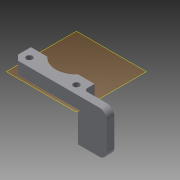
# Autodesk Inventor part: RightBracket
Saved by Autodesk Inventor 2014 SP1 (Build 180222100, 222)
## iProperties
Created: 2017-02-10
Part Number: RightBracket
Material: Generic
Document SubType Name: Modeling
Designer: danielsikar
Density: 1 g/cm^3
Appearance: Default
d0: 12.000 mm
d1: 12.000 mm
d2: 8.000 mm
d3: 0.00 deg
d4: 8.000 mm
d5: 5.000 mm
d6: 20.000 mm
d7: 0.00 deg
d8: 19.000 mm
d9: 5.000 mm
d10: 20.000 mm
d11: 0.00 deg
d14: 2.000 mm
d15: 0.500 mm
d16: 8.000 mm
d17: 0.00 deg
Author: danielsikar
Autodesk Inventor part; units mm, degrees
ref_plane "YZ Plane" through (0, 0, 0) normal (1, 0, 0) x (0, 1, 0)
ref_plane "XZ Plane" through (0, 0, 0) normal (0, 1, 0) x (-1, 0, 0)
ref_plane "XY Plane" through (0, 0, 0) normal (0, 0, 1) x (1, 0, 0)
ref_plane "Work Plane1" through (21, 21, 47) normal (0, 0, 1) x (1, 0, 0)
sketch "Sketch1" plane through (21, 21, 47) normal (0, 0, 1) x (1, 0, 0)
  line L0 (21, -17.5) -> (21, 17.5) construction
  line L1 (-17.5, -21) -> (17.5, -21) construction
  line L2 (21, -21) -> (9, -21)
  line L3 (9, -21) -> (9, -9)
  line L4 (9, -9) -> (21, -9)
  line L5 (21, -9) -> (21, -21)
  point P0 (-21, -21)
  dimension "d0" = 12
  dimension "d1" = 12
  constraints: 8 end point, 2 parallel, 1 horizontal, 1 perpendicular, 1 point on line
  measures "d0" distance of L3.end L4.end
  measures "d1" distance of L2.end L3.end
extrude "Extrusion1" add sketch "Sketch1" along normal blind 8
sketch "Sketch2" plane through (42, 0, 47) normal (1, 0, 0) x (0, 0, -1)
  line L0 (-8, 0) -> (0, 0)
  line L1 (0, 0) -> (0, 5)
  line L2 (0, 5) -> (-8, 5)
  line L3 (-8, 5) -> (-8, 0)
  point P0 (47, 0)
  dimension "d4" = 8
  dimension "d5" = 5
  constraints: 8 end point, 2 parallel, 1 horizontal, 1 perpendicular
  measures "d4" distance of L2.end L1.end
  measures "d5" distance of L1.end L0.end
extrude "Extrusion2" add sketch "Sketch2" along normal blind 20
sketch "Sketch3" plane through (21, 21, 47) normal (0, 0, -1) x (-1, 0, 0)
  line L0 (-41, -16) -> (-22, -16)
  line L1 (-22, -16) -> (-22, -21)
  line L2 (-22, -21) -> (-41, -21)
  line L3 (-41, -21) -> (-41, -16)
  point P0 (21, -21)
  dimension "d8" = 19
  dimension "d9" = 5
  constraints: 8 end point, 2 parallel, 1 horizontal, 1 perpendicular
  measures "d8" distance of L1.end L2.end
  measures "d9" distance of L0.end L1.end
extrude "Extrusion3" add sketch "Sketch3" along normal blind 20
fillet "Fillet3" radius 2 1 edges at (42, 5, 51)
sketch "Sketch4" plane through (21, 21, 55) normal (0, 0, 1) x (1, 0, 0)
  circle A0 centre (15.5, -15.5) radius 1.5 projected
  circle A1 centre (15.5, -15.5) radius 2
  point P0 (-21, -21)
  dimension "d15" = 0.5
  constraints: 1 centre point
  measures "d15" radial gap between concentric circles of A1 A0
extrude "Extrusion4" cut sketch "Sketch4" against normal blind 8 contours A0 | A1
sketch "Sketch5" plane through (30, 0, 47) normal (-1, 0, 0) x (0, 0, 1)
  line L0 (0, 0) -> (0, 12) projected
  line L1 (0, 0) -> (8, 0) projected
  line L2 (8, 12) -> (8, 0) projected
  line L3 (0, 12) -> (8, 12) projected
  point P0 (-47, 0)
ref_plane "Work Plane2" through (0, 3.5, 0) normal (-1, 0, 0) x (0, 0, 1)
extrude "Extrusion5" add sketch "Sketch5" along normal up to surface (30 mm away)
sketch "Sketch6" plane through (21, 21, 55) normal (0, 0, 1) x (1, 0, 0)
  circle A0 centre (-15.5, -15.5) radius 1.5 projected
  circle A1 centre (-15.5, -15.5) radius 2
  dimension "d20" = 0.5
  constraints: 1 centre point
  measures "d20" radial gap between concentric circles of A1 A0
extrude "Extrusion6" cut sketch "Sketch6" against normal blind 8 contours A0 | A1
sketch "Sketch7" plane through (21, 21, 55) normal (0, 0, 1) x (1, 0, 0)
  line L0 (21, -9) -> (-21, -9) projected
  circle A0 centre (0, 0) radius 11 projected
  arc A1 (-10.1679, -9) -> (10.1679, -9) centre (0, 0) ccw
  line L1 (-10.1679, -9) -> (11.2714, -9)
  line L2 (-13.5789, -9) -> (17.965, -9)
  constraints: 6 point on line, 4 end point, 2 point on circle, 1 centre point
extrude "Extrusion7" cut sketch "Sketch7" against normal blind 8 contours A1 L0 A0 | A0 L0 picked at (-1.3175, -9.4218)
sketch "Sketch8" plane through (21, 21, 55) normal (0, 0, 1) x (1, 0, 0)
  line L0 (-21, -9) -> (-21, -21) projected
  line L1 (41, -21) -> (-21, -21) projected
  line L2 (-17.5, -21) -> (-21, -17.5) projected
extrude "Extrusion8" cut sketch "Sketch8" against normal blind 8
fillet "Fillet4" radius 5 2 edges at (62, 2.5, 55) (62, 2.5, 27)
body "Solid1"
